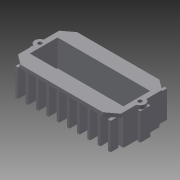
# Autodesk Inventor part: power channel
Saved by Autodesk Inventor 2014 SP1 (Build 180222100, 222)
## iProperties
Created: 2017-07-21
Part Number: power channel
Material: Generic
Document SubType Name: Modeling
Designer: kteo17
Density: 1 g/cm^3
Appearance: Default
Author: kteo17
Autodesk Inventor part; units mm, degrees
ref_plane "YZ Plane" through (0, 0, 0) normal (1, 0, 0) x (0, 1, 0)
ref_plane "XZ Plane" through (0, 0, 0) normal (0, 1, 0) x (-1, 0, 0)
ref_plane "XY Plane" through (0, 0, 0) normal (0, 0, 1) x (1, 0, 0)
sketch "Sketch1" plane through (0, 0, 0) normal (0, 0, 1) x (1, 0, 0)
  line L0 (0, 0) -> (63.5, 0)
  line L1 (63.5, 0) -> (63.5, 22.225)
  line L2 (63.5, 22.225) -> (0, 22.225)
  line L3 (0, 22.225) -> (0, 0)
  dimension "d0" = 63.5
  dimension "d1" = 22.225
  constraints: 8 end point, 2 parallel, 1 horizontal, 1 perpendicular
  measures "d0" distance of L2.end L1.end
  measures "d1" distance of L1.end L0.end
extrude "Extrusion1" add sketch "Sketch1" along normal blind 2.54
sketch "Sketch2" plane through (0, 0, 2.54) normal (0, 0, 1) x (1, 0, 0)
  line L0 (0, 0) -> (63.5, 0) projected
  line L1 (63.5, 0) -> (63.5, 22.225) projected
  line L2 (63.5, 22.225) -> (0, 22.225) projected
  line L3 (0, 22.225) -> (0, 0) projected
  line L4 (3.175, 19.685) -> (60.325, 19.685)
  line L5 (60.325, 2.54) -> (3.175, 2.54)
  line L6 (3.175, 19.685) -> (3.175, 2.54)
  line L7 (60.325, 19.685) -> (60.325, 2.54)
  dimension "d4" = 2.54
  dimension "d43" = 2.54
  constraints: 8 end point, 2 perpendicular
  measures "d4" distance between parallel lines of L2 L4
  measures "d43" distance between parallel lines of L0 L5
extrude "Extrusion2" add sketch "Sketch2" along normal blind 16.51
sketch "Sketch3" plane through (0, 0, 0) normal (0, 0, -1) x (-1, 0, 0)
  line L0 (-63.5, 0) -> (-63.5, 22.225) projected
  line L1 (-63.5, 14.2875) -> (-58.7375, 14.2875)
  line L2 (-58.7375, 14.2875) -> (-58.7375, 7.9375)
  line L3 (-58.7375, 7.9375) -> (-63.5, 7.9375)
  line L4 (-63.5, 7.9375) -> (-63.5, 14.2875)
  constraints: 8 end point, 2 parallel, 1 horizontal, 1 perpendicular, 1 point on line
extrude "Extrusion3" cut sketch "Sketch3" against normal blind 5.08
sketch "Sketch17" plane through (0, 0, 19.05) normal (0, 0, 1) x (1, 0, 0)
  line L0 (0, 22.225) -> (0, 0) projected
  line L1 (63.5, 0) -> (63.5, 22.225) projected
  arc A0 (63.5, 12.0042) -> (63.5, 10.2208) centre (62.7063, 11.1125) ccw projected
  line L2 (63.5, 0) -> (63.5, 22.225) projected
  line L3 (0, 22.225) -> (0, 0) projected
  arc A1 (0, 14.1867) -> (0, 8.0383) centre (0.7937, 11.1125) ccw
  arc A2 (63.5, 8.0383) -> (63.5, 14.1867) centre (62.7063, 11.1125) ccw
  arc A3 (0, 10.2208) -> (0, 12.0042) centre (0.7937, 11.1125) ccw
  arc A4 (63.5, 12.0042) -> (63.5, 10.2208) centre (62.7063, 11.1125) ccw
  line L4 (0, 12.0042) -> (0, 10.2208)
  line L5 (63.5, 12.0042) -> (63.5, 10.2208)
  constraints: 9 point on circle, 8 point on line, 4 centre point, 4 end point, 3 coincident, 1 parallel
extrude "Extrusion15" add sketch "Sketch17" against normal blind 2.2225 contours L0 A1 | L1 A2
sketch "Sketch18" plane through (0, 0, 19.05) normal (0, 0, 1) x (1, 0, 0)
  arc A0 (63.5, 8.0383) -> (63.5, 14.1867) centre (62.7063, 11.1125) ccw projected
  arc A1 (0, 14.1867) -> (0, 8.0383) centre (0.7937, 11.1125) ccw projected
  circle A2 centre (0.7937, 11.1125) radius 1.1938
  circle A3 centre (62.7063, 11.1125) radius 1.1938
  dimension "d46" = 2.3876
  constraints: 2 centre point, 2 coincident
  measures "d46" diameter of A2
extrude "Extrusion16" cut sketch "Sketch18" against normal blind 2.032
sketch "Sketch19" plane through (0, 0, 5.08) normal (0, 0, -1) x (-1, 0, 0)
  line L0 (-60.325, 14.2875) -> (-60.325, 7.9375) projected
  line L1 (-63.5, 10.2213) -> (-60.325, 10.2213)
  line L2 (-60.325, 10.2213) -> (-60.325, 12.0037)
  line L3 (-60.325, 12.0037) -> (-63.5, 12.0037)
  line L4 (-63.5, 12.0037) -> (-63.5, 10.2213)
  line L5 (-63.5, 10.2213) -> (-60.325, 12.0037) construction
  line L6 (-60.325, 10.2213) -> (-63.5, 12.0037) construction
  point P0 (0, 0)
  point P1 (-61.9125, 11.1125)
  constraints: 12 end point, 2 midpoint, 2 parallel, 1 horizontal, 1 perpendicular, 1 point on line
extrude "Extrusion17" add sketch "Sketch19" along normal blind 5.08
sketch "Sketch20" plane through (63.5, 0, 19.05) normal (1, 0, 0) x (0, 0, -1)
  line L0 (13.97, 10.2213) -> (19.05, 10.2213) projected
  line L1 (13.97, 12.0037) -> (14.224, 12.0037)
  line L2 (14.224, 12.0037) -> (14.224, 10.2213)
  line L3 (14.224, 10.2213) -> (13.97, 10.2213)
  line L4 (13.97, 10.2213) -> (13.97, 12.0037)
  dimension "d51" = 0.254
  constraints: 8 end point, 2 parallel, 1 horizontal, 1 perpendicular, 1 point on line
  measures "d51" distance of L2.end L3.end
extrude "Extrusion18" cut sketch "Sketch20" against normal blind 3.175
sketch "Sketch21" plane through (0, 0, 16.8275) normal (0, 0, -1) x (-1, 0, 0)
  line L0 (2.427, 14.1867) -> (0.8395, 14.1867)
  line L1 (0.8395, 14.1867) -> (0.8395, 8.0383)
  line L2 (0.8395, 8.0383) -> (2.427, 8.0383)
  line L3 (2.427, 8.0383) -> (2.427, 14.1867)
  line L4 (-65.927, 8.0383) -> (-64.3395, 8.0383)
  line L5 (-64.3395, 8.0383) -> (-64.3395, 14.1867)
  line L6 (-64.3395, 14.1867) -> (-65.927, 14.1867)
  line L7 (-65.927, 14.1867) -> (-65.927, 8.0383)
  point P0 (0, 0)
  constraints: 16 end point, 4 parallel, 2 horizontal, 2 perpendicular
extrude "Extrusion19" add sketch "Sketch21" along normal blind 16.8275
sketch "Sketch22" plane through (0, 0, 19.05) normal (0, 0, 1) x (1, 0, 0)
  line L0 (0, 22.225) -> (63.5, 22.225)
  line L1 (63.5, 22.225) -> (63.5, 23.8125)
  line L2 (57.15, 28.575) -> (6.35, 28.575)
  line L3 (0, 23.8125) -> (0, 22.225)
  line L4 (0, 0) -> (63.5, 0)
  line L5 (63.5, 0) -> (63.5, -1.5875)
  line L6 (57.15, -6.35) -> (6.35, -6.35)
  line L7 (0, -1.5875) -> (0, 0)
  line L8 (0, 23.8125) -> (6.35, 28.575)
  line L9 (63.5, 23.8125) -> (57.15, 28.575)
  line L10 (0, -1.5875) -> (6.35, -6.35)
  line L11 (63.5, -1.5875) -> (57.15, -6.35)
  dimension "d56" = 34.925
  constraints: 24 end point, 6 parallel, 2 horizontal, 2 perpendicular
  measures "d56" distance between parallel lines of L6 L2
extrude "Extrusion20" add sketch "Sketch22" against normal blind 2.2225
sketch "Sketch23" plane through (0, 0, 16.8275) normal (0, 0, -1) x (-1, 0, 0)
  line L0 (-6.35, 28.575) -> (-57.15, 28.575) projected
  line L1 (-60.325, 28.575) -> (-58.7375, 28.575)
  line L2 (-58.7375, 28.575) -> (-58.7375, 23.8125)
  line L3 (-58.7375, 23.8125) -> (-60.325, 23.8125)
  line L4 (-60.325, 23.8125) -> (-60.325, 28.575)
  line L5 (-53.975, 28.575) -> (-52.3875, 28.575)
  line L6 (-52.3875, 28.575) -> (-52.3875, 23.8125)
  line L7 (-52.3875, 23.8125) -> (-53.975, 23.8125)
  line L8 (-53.975, 23.8125) -> (-53.975, 28.575)
  line L9 (-47.625, 28.575) -> (-46.0375, 28.575)
  line L10 (-46.0375, 28.575) -> (-46.0375, 23.8125)
  line L11 (-46.0375, 23.8125) -> (-47.625, 23.8125)
  line L12 (-47.625, 23.8125) -> (-47.625, 28.575)
  line L13 (-41.275, 28.575) -> (-39.6875, 28.575)
  line L14 (-39.6875, 28.575) -> (-39.6875, 23.8125)
  line L15 (-39.6875, 23.8125) -> (-41.275, 23.8125)
  line L16 (-41.275, 23.8125) -> (-41.275, 28.575)
  line L17 (-34.925, 28.575) -> (-33.3375, 28.575)
  line L18 (-33.3375, 28.575) -> (-33.3375, 23.8125)
  line L19 (-33.3375, 23.8125) -> (-34.925, 23.8125)
  line L20 (-34.925, 23.8125) -> (-34.925, 28.575)
  line L21 (-28.575, 28.575) -> (-26.9875, 28.575)
  line L22 (-26.9875, 28.575) -> (-26.9875, 23.8125)
  line L23 (-26.9875, 23.8125) -> (-28.575, 23.8125)
  line L24 (-28.575, 23.8125) -> (-28.575, 28.575)
  line L25 (-22.225, 28.575) -> (-20.6375, 28.575)
  line L26 (-20.6375, 28.575) -> (-20.6375, 23.8125)
  line L27 (-20.6375, 23.8125) -> (-22.225, 23.8125)
  line L28 (-22.225, 23.8125) -> (-22.225, 28.575)
  line L29 (-15.875, 28.575) -> (-14.2875, 28.575)
  line L30 (-14.2875, 28.575) -> (-14.2875, 23.8125)
  line L31 (-14.2875, 23.8125) -> (-15.875, 23.8125)
  line L32 (-15.875, 23.8125) -> (-15.875, 28.575)
  line L33 (-9.525, 28.575) -> (-7.9375, 28.575)
  line L34 (-7.9375, 28.575) -> (-7.9375, 23.8125)
  line L35 (-7.9375, 23.8125) -> (-9.525, 23.8125)
  line L36 (-9.525, 23.8125) -> (-9.525, 28.575)
  line L37 (-3.175, 28.575) -> (-1.5875, 28.575)
  line L38 (-1.5875, 28.575) -> (-1.5875, 23.8125)
  line L39 (-1.5875, 23.8125) -> (-3.175, 23.8125)
  line L40 (-3.175, 23.8125) -> (-3.175, 28.575)
  line L41 (-60.325, -6.35) -> (-58.7375, -6.35)
  line L42 (-58.7375, -6.35) -> (-58.7375, -1.5875)
  line L43 (-58.7375, -1.5875) -> (-60.325, -1.5875)
  line L44 (-60.325, -1.5875) -> (-60.325, -6.35)
  line L45 (-53.975, -6.35) -> (-52.3875, -6.35)
  line L46 (-52.3875, -6.35) -> (-52.3875, -1.5875)
  line L47 (-52.3875, -1.5875) -> (-53.975, -1.5875)
  line L48 (-53.975, -1.5875) -> (-53.975, -6.35)
  line L49 (-47.625, -6.35) -> (-46.0375, -6.35)
  line L50 (-46.0375, -6.35) -> (-46.0375, -1.5875)
  line L51 (-46.0375, -1.5875) -> (-47.625, -1.5875)
  line L52 (-47.625, -1.5875) -> (-47.625, -6.35)
  line L53 (-41.275, -6.35) -> (-39.6875, -6.35)
  line L54 (-39.6875, -6.35) -> (-39.6875, -1.5875)
  line L55 (-39.6875, -1.5875) -> (-41.275, -1.5875)
  line L56 (-41.275, -1.5875) -> (-41.275, -6.35)
  line L57 (-34.925, -6.35) -> (-33.3375, -6.35)
  line L58 (-33.3375, -6.35) -> (-33.3375, -1.5875)
  line L59 (-33.3375, -1.5875) -> (-34.925, -1.5875)
  line L60 (-34.925, -1.5875) -> (-34.925, -6.35)
  line L61 (-28.575, -6.35) -> (-26.9875, -6.35)
  line L62 (-26.9875, -6.35) -> (-26.9875, -1.5875)
  line L63 (-26.9875, -1.5875) -> (-28.575, -1.5875)
  line L64 (-28.575, -1.5875) -> (-28.575, -6.35)
  line L65 (-22.225, -6.35) -> (-20.6375, -6.35)
  line L66 (-20.6375, -6.35) -> (-20.6375, -1.5875)
  line L67 (-20.6375, -1.5875) -> (-22.225, -1.5875)
  line L68 (-22.225, -1.5875) -> (-22.225, -6.35)
  line L69 (-15.875, -6.35) -> (-14.2875, -6.35)
  line L70 (-14.2875, -6.35) -> (-14.2875, -1.5875)
  line L71 (-14.2875, -1.5875) -> (-15.875, -1.5875)
  line L72 (-15.875, -1.5875) -> (-15.875, -6.35)
  line L73 (-9.525, -6.35) -> (-7.9375, -6.35)
  line L74 (-7.9375, -6.35) -> (-7.9375, -1.5875)
  line L75 (-7.9375, -1.5875) -> (-9.525, -1.5875)
  line L76 (-9.525, -1.5875) -> (-9.525, -6.35)
  line L77 (-3.175, -6.35) -> (-1.5875, -6.35)
  line L78 (-1.5875, -6.35) -> (-1.5875, -1.5875)
  line L79 (-1.5875, -1.5875) -> (-3.175, -1.5875)
  line L80 (-3.175, -1.5875) -> (-3.175, -6.35)
  point P0 (0, 0)
  constraints: 160 end point, 40 parallel, 20 horizontal, 20 perpendicular, 9 other
extrude "Extrusion21" add sketch "Sketch23" along normal blind 16.8275
body "Solid1"
